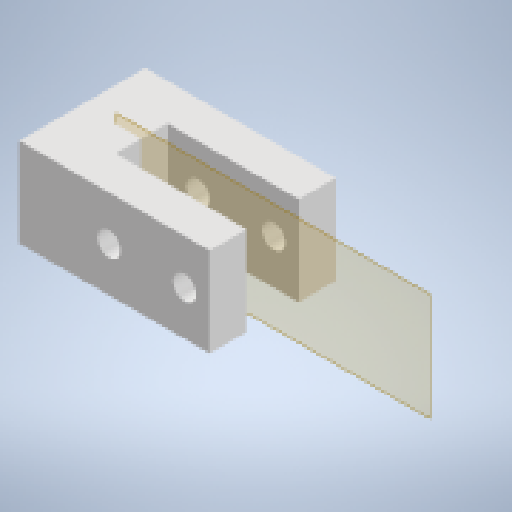
# Autodesk Inventor part: pinzatula1
Saved by Autodesk Inventor 2024.3 (Build 283343000, 343)
## iProperties
Created: 2025-07-08
Part Number: pinzatula1
Material: ABS Plastic
Document SubType Name: Modeling
Designer: user
Density: 1.06 g/cm^3
Appearance: Smooth - White
Author: user
Autodesk Inventor part; units mm, degrees
ref_plane "YZ Plane" through (0, 0, 0) normal (1, 0, 0) x (0, 1, 0)
ref_plane "XZ Plane" through (0, 0, 0) normal (0, 1, 0) x (-1, 0, 0)
ref_plane "XY Plane" through (0, 0, 0) normal (0, 0, 1) x (1, 0, 0)
sketch "Sketch1" plane through (0, 0, 0) normal (0, 0, 1) x (1, 0, 0)
  circle A0 centre (14.1, 6) radius 1.6 projected
  circle A1 centre (3.9, 6) radius 1.6 projected
  line L0 (0, 0) -> (35, 0) projected
  line L1 (35, 0) -> (35, 12) projected
  line L2 (0, 12) -> (35, 12) projected
  line L3 (0, 0) -> (0, 12) projected
  line L4 (17.5, 0) -> (17.5, 12)
  constraints: 2 end point, 2 midpoint
ref_plane "Work Plane1" through (0, 12, -3.5) normal (0, 0, 1) x (1, 0, 0)
extrude "Extrusion1" add sketch "Sketch1" along normal blind 5 contours L3 L2 L4 L0
mirror "Mirror1" about plane through (0, 12, -3.5) normal (0, 0, 1) of "Extrusion1"
sketch "Sketch2" plane through (0, 0, -7) normal (-1, 0, 0) x (0, 0, 1)
  line L0 (0, 12) -> (0, 0) projected
  line L1 (0, 12) -> (-5, 12) projected
  line L2 (-5, 12) -> (-5, 0) projected
  line L3 (0, 0) -> (-5, 0) projected
  line L4 (10.85, 12) -> (10.85, 0) projected
  line L5 (7, 12) -> (7, 0) projected
  line L6 (7, 0) -> (12, 0) projected
  line L7 (12, 12) -> (12, 0) projected
  line L8 (7, 12) -> (12, 12) projected
extrude "Extrusion2" add sketch "Sketch2" along normal blind 0.2
sketch "Sketch3" plane through (-0.2, 0, -7) normal (-1, 0, 0) x (0, 0, 1)
  line L0 (-5, 0) -> (0, 0) projected
  line L1 (0, 0) -> (0, 12) projected
  line L2 (0, 12) -> (-5, 12) projected
  line L3 (-5, 12) -> (-5, 0) projected
  line L4 (10.85, 12) -> (10.85, 0) projected
  line L5 (7, 0) -> (12, 0) projected
  line L6 (12, 0) -> (12, 12) projected
  line L7 (12, 12) -> (7, 12) projected
  line L8 (7, 12) -> (7, 0) projected
  line L9 (-5, 12) -> (12, 12)
  line L10 (12, 12) -> (12, 0)
  line L11 (12, 0) -> (-5, 0)
  line L12 (-5, 0) -> (-5, 12)
  constraints: 8 end point, 2 parallel, 1 horizontal, 1 perpendicular
extrude "Extrusion3" add sketch "Sketch3" along normal blind 8
ref_plane "Work Plane2" through (-58.2, 0, -7) normal (-1, 0, 0) x (0, 0, 1)
sketch "Sketch4" plane through (-58.2, 0, -7) normal (-1, 0, 0) x (0, 0, 1)
  line L0 (-5, 0) -> (12, 0) projected
  line L1 (12, 0) -> (12, 12) projected
  line L2 (12, 12) -> (-5, 12) projected
  line L3 (-5, 12) -> (-5, 0) projected
  line L4 (3.5, 0) -> (38.5, 0) construction
  line L5 (36.7487, 51.7487) -> (19.7487, 51.7487)
  line L6 (19.7487, 51.7487) -> (19.7487, 39.7487)
  line L7 (19.7487, 39.7487) -> (36.7487, 39.7487)
  line L8 (36.7487, 39.7487) -> (36.7487, 51.7487)
  line L9 (36.7487, 51.7487) -> (19.7487, 39.7487) construction
  line L10 (19.7487, 51.7487) -> (36.7487, 39.7487) construction
  point P0 (7, 0)
  point P1 (28.2487, 45.7487)
  point P2 (28.2487, 45.7487)
  dimension "d9" = 17
  dimension "d10" = 12
  dimension "d16" = 45.7487
  dimension "d17" = 16.2487
  constraints: 14 end point, 3 midpoint, 2 horizontal, 2 parallel, 1 perpendicular
  measures "d9" distance of L7.end L6.end
  measures "d10" distance of L6.end L5.end
  measures "d16" distance from line of L4 point (28.249, 45.749)
  measures "d17" distance from line of L1 point (28.249, 45.749)
sketch "Sketch5" plane through (-8.2, 0, -7) normal (-1, 0, 0) x (0, 0, 1)
  line L0 (-5, 0) -> (12, 0) projected
  line L1 (12, 0) -> (12, 12) projected
  line L2 (12, 12) -> (-5, 12) projected
  line L3 (-5, 12) -> (-5, 0) projected
  point P0 (7, 0)
loft "Loft1" add profiles "Sketch4" section 1 edges at (-8.2, 0, -3.5) (-8.2, 6, 5) (-8.2, 12, -3.5) (-8.2, 6, -12) contours L8 L7 L6 L5
sketch "Sketch6" plane through (-58.2, 39.7487, 29.7487) normal (-1, 0, 0) x (0, 0, 1)
  line L0 (0, 0) -> (-17, 0) projected
  line L1 (0, 12) -> (0, 0) projected
  line L2 (-17, 12) -> (0, 12) projected
  line L3 (-17, 0) -> (-17, 12) projected
  point P0 (-29.7487, -39.7487)
ref_plane "Work Plane3" through (-58.2, 45.7487, 29.7487) normal (0, 1, 0) x (1, 0, 0)
sketch "Sketch7" plane through (-58.2, 45.7487, 29.7487) normal (0, 1, 0) x (1, 0, 0)
  line L0 (0, 0) -> (0, 17) projected
  arc A0 (-113.5209, 8.5) -> (0, 8.5) centre (-56.7605, 64.8014) ccw
  point P0 (58.2, 29.7487)
  constraints: 2 point on circle, 1 centre point, 1 midpoint
sweep "Sweep1" add profiles "Sketch6" path "Sketch7" path curves A0
sketch "Sketch8" plane through (-58.2, 39.7487, 12.7487) normal (0, -1, 0) x (1, 0, 0)
  arc A0 (0, 0) -> (-105.0212, 8.569) centre (-56.7605, -47.8014) ccw projected
  point P0 (58.2, -12.7487)
sketch "Sketch9" plane through (-58.2, 51.7487, 29.7487) normal (0, 1, 0) x (1, 0, 0)
  arc A0 (-105.0212, 8.431) -> (0, 17) centre (-56.7605, 64.8014) ccw projected
  line L0 (-105.0212, 8.431) -> (-121.9115, 22.0076)
  line L1 (-121.9115, 22.0076) -> (-122.1671, 29.7487)
  line L2 (-122.1671, 29.7487) -> (0, 29.7487)
  line L3 (0, 29.7487) -> (0, 17)
  point P0 (58.2, 29.7487)
  constraints: 8 end point, 1 horizontal, 1 perpendicular
extrude "Extrusion4" add sketch "Sketch9" against normal blind 8
chamfer "Chamfer1" distance 22 distance2 8 1 edges at (-119.2836, 43.7487, 0) measured on face at (-119.2836, 43.7487, 0.5)
sketch "Sketch10" plane through (-58.2, 39.7487, 12.7487) normal (0, -1, 0) x (1, 0, 0)
  arc A0 (0, 0) -> (-105.0212, 8.569) centre (-56.7605, -47.8014) ccw projected
  arc A1 (3.0596, 2.5766) -> (-107.6226, 11.6076) centre (-56.7605, -47.8014) ccw
  line L0 (-105.0212, 8.569) -> (-122.0206, 8.431) projected
  line L1 (-105.0212, 8.569) -> (-107.6226, 11.6076)
  line L2 (0, 0) -> (0, 17) projected
  line L3 (0, 6.0004) -> (0, 0)
  point P0 (58.2, -12.7487)
  dimension "d25" = 4
  constraints: 4 end point, 3 point on circle, 1 centre point, 1 collinear
  measures "d25" radial gap between concentric circles of A0 A1
extrude "Extrusion5" add sketch "Sketch10" along normal blind 20
sketch "Sketch11" plane through (-58.2, 19.7487, 12.7487) normal (0, -1, 0) x (1, 0, 0)
  arc A0 (0, 0) -> (-105.0212, 8.569) centre (-56.7605, -47.8014) ccw projected
  line L0 (0, 0) -> (0, 6.0004) projected
  arc A1 (0, 6.0004) -> (-107.6226, 11.6076) centre (-56.7605, -47.8014) ccw projected
  line L1 (-107.6226, 11.6076) -> (-105.0212, 8.569) projected
  line L2 (-107.6226, 11.6076) -> (-107.4924, -4.4259)
  line L3 (-122.0206, 8.431) -> (-105.0212, 8.569) projected
  line L4 (0, -3.553) -> (0, 3.5909)
  arc A2 (0, -3.553) -> (-107.4924, -4.4259) centre (-52.5715, -148.6478) ccw
  point P0 (58.2, -12.7487)
  point P1 (0, 0)
  point P2 (-107.5977, 8.5481)
  constraints: 4 end point, 2 point on circle, 1 centre point, 1 perpendicular, 1 point on line
extrude "Extrusion6" add sketch "Sketch11" along normal blind 3 contours L4 A2 L2 L3 A0 | A0 L1 A1 L0
body "Solid1"
